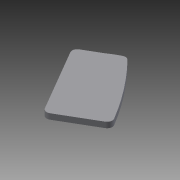
# Autodesk Inventor part: adelante
Saved by Autodesk Inventor 2015 (Build 190159000, 159)
## iProperties
Created: 2017-10-04
Part Number: adelante
Material: Generic
Document SubType Name: Modeling
Designer: Max
Density: 1 g/cm^3
Appearance: Default
Author: Max
Autodesk Inventor part; units mm, degrees
ref_plane "YZ Plane" through (0, 0, 0) normal (1, 0, 0) x (0, 1, 0)
ref_plane "XZ Plane" through (0, 0, 0) normal (0, 1, 0) x (-1, 0, 0)
ref_plane "XY Plane" through (0, 0, 0) normal (0, 0, 1) x (1, 0, 0)
sketch "Sketch1" plane through (0, 0, 0) normal (0, 0, 1) x (1, 0, 0)
  line L0 (-20.4878, 268.8466) -> (-13.846, 272.7251)
  line L1 (-9.0847, 275.4971) -> (-3.3614, 279.1755)
  line L2 (-20.4878, 268.8466) -> (-29.1232, 263.8039)
  line L3 (-3.3614, 279.1755) -> (5.4134, 283.9717)
  arc A0 (54.3957, 219.9337) -> (5.4134, 283.9717) centre (-211.5069, 67.2983) ccw
  line L4 (11.1931, 194.7636) -> (22.5933, 201.4009)
  line L5 (44.4637, 214.1339) -> (54.3957, 219.9337)
  line L6 (-29.1232, 263.8039) -> (1.9667, 210.5634)
  line L7 (4.4628, 206.2891) -> (11.1931, 194.7636)
  line L8 (-13.846, 272.7251) -> (-9.0847, 275.4971)
  line L9 (44.4637, 214.1339) -> (22.5933, 201.4009)
  line L10 (4.4628, 206.2891) -> (1.9667, 210.5634)
  point P0 (0, 0)
  dimension "d0" = 20
  dimension "d2" = 10
  dimension "d4" = 50
  dimension "d5" = 10
  constraints: 22 end point, 2 perpendicular, 2 point on circle, 1 centre point, 1 collinear, 1 parallel
  measures "d0" distance of L2.start L1.end
  measures "d2" distance of L2.start L6.start
  measures "d4" distance of L4.start L5.end
  measures "d5" distance of L1.end L3.end
extrude "Extrusion1" add sketch "Sketch1" along normal blind 5.5
fillet "Fillet1" radius 5 4 edges at (5.4134, 283.9717, 2.75) (54.3957, 219.9337, 2.75) (11.1931, 194.7636, 2.75) (-29.1232, 263.8039, 2.75)
body "Solid1"
